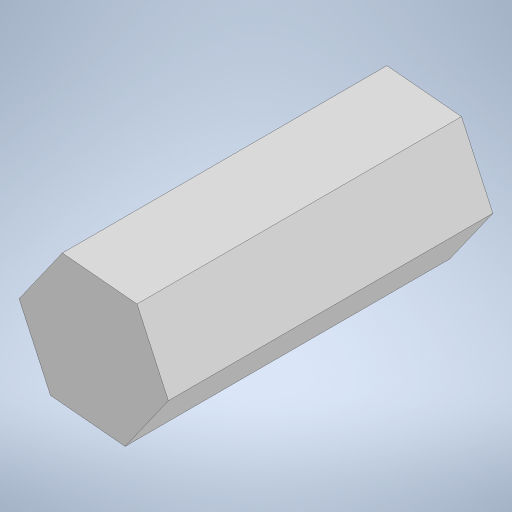
# Autodesk Inventor part: 4-bar intake peg
Saved by Autodesk Inventor 2023 (Build 270158030, 158C)
## iProperties
Created: 2022-07-19
Part Number: 4-bar intake peg
Material: Generic
Document SubType Name: Modeling
Designer: rm0990889
Density: 1 g/cm^3
Appearance: Default
Author: rm0990889
Autodesk Inventor part; units mm, degrees
ref_plane "YZ Plane" through (0, 0, 0) normal (1, 0, 0) x (0, 1, 0)
ref_plane "XZ Plane" through (0, 0, 0) normal (0, 1, 0) x (-1, 0, 0)
ref_plane "XY Plane" through (0, 0, 0) normal (0, 0, 1) x (1, 0, 0)
sketch "Sketch1" plane through (0, 0, 0) normal (0, 0, 1) x (1, 0, 0)
  circle A0 centre (0, 0) radius 6.35
  line L0 (7.3015, -0.672) -> (3.0688, -6.6593)
  line L1 (3.0688, -6.6593) -> (-4.2327, -5.9873)
  line L2 (-4.2327, -5.9873) -> (-7.3015, 0.672)
  line L3 (-7.3015, 0.672) -> (-3.0688, 6.6593)
  line L4 (-3.0688, 6.6593) -> (4.2327, 5.9873)
  line L5 (4.2327, 5.9873) -> (7.3015, -0.672)
  point P0 (5.7671, 2.6576)
  dimension "d0" = 12.7
  constraints: 12 end point, 2 coincident, 1 midpoint, 16 other
extrude "Extrusion1" add sketch "Sketch1" along normal blind 31.75
body "Solid1"
